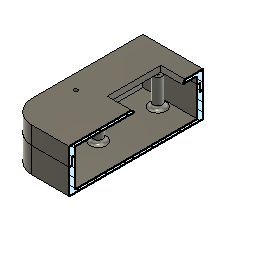
ReceiverCase (Autodesk Fusion 360 design; units mm, degrees)
Autodesk Fusion 360 part; units mm, degrees
sketch "Sketch1" plane through (0, 0, 0) normal (0, 1, 0) x (1, 0, 0)
  line L0 (22.5, 22.5) -> (-22.5, 22.5)
  line L1 (-22.5, 22.5) -> (-22.5, -22.5)
  line L2 (-22.5, -22.5) -> (22.5, -22.5)
  line L3 (22.5, -22.5) -> (22.5, 22.5)
  line L4 (22.5, 22.5) -> (-22.5, -22.5) construction
  line L5 (-22.5, 22.5) -> (22.5, -22.5) construction
  circle A0 centre (-20, 20) radius 1
  circle A1 centre (20, 20) radius 1
  circle A2 centre (20, -20) radius 1
  circle A3 centre (-20, -20) radius 1
  line L6 (-13.9694, -16) -> (-13.9694, 16)
  line L7 (-13.9694, 16) -> (7.9088, 16)
  line L8 (7.9088, 16) -> (7.9088, -16)
  line L9 (7.9088, -16) -> (-13.9694, -16)
  line L10 (25, -29.5) -> (-25, -29.5)
  line L11 (-25, -29.5) -> (-25, -54.5)
  line L12 (-25, -54.5) -> (25, -54.5)
  line L13 (25, -54.5) -> (25, -29.5)
  line L14 (25, -29.5) -> (-25, -54.5) construction
  line L15 (-25, -29.5) -> (25, -54.5) construction
  line L16 (30, 30) -> (-40, 30)
  line L17 (-40, 30) -> (-40, -60)
  line L18 (-40, -60) -> (30, -60)
  line L19 (30, -60) -> (30, 30)
  arc A4 (30, 22.5) -> (22.5, 30) centre (22.5, 22.5) ccw
  arc A5 (-40, -44) -> (-25, -60) centre (-23.9667, -44) ccw
  arc A6 (25, -60) -> (30, -55) centre (25, -55) ccw
  circle A7 centre (-20, 20) radius 3
  circle A8 centre (20, 20) radius 3
  circle A9 centre (20, -20) radius 3
  circle A10 centre (-20, -20) radius 3
  dimension "d1" = 45
  dimension "d2" = 45
  dimension "d9" = 50
  dimension "d10" = 25
extrude "Extrude1" add sketch "Sketch1" along normal blind 1 contours L0 L3 A8 | L0 L3 A8 | L0 L1 L2 L3 A7 A8 A9 A10 | L0 L1 A7 | L2 L3 A9 | L0 L1 A7 | L2 L3 A9 | L1 L2 A10 | L1 L2 A10 | L6 L7 L8 L9 makes body 1
extrude "Extrude2" add sketch "Sketch1" along normal blind 6 contours L6 L7 L8 L9 bodies 1
extrude "Extrude3" add sketch "Sketch1" along normal blind 20 separate body contours L10 L11 L12 L13 makes body 2
sketch "Sketch2" plane through (0, 0, 0) normal (0, 1, 0) x (1, 0, 0)
  arc A0 (30, 22.5) -> (22.5, 30) centre (22.5, 22.5) ccw
  line L0 (-40, 30) -> (22.5, 30)
  line L1 (30, 22.5) -> (30, -55)
  arc A1 (25, -60) -> (30, -55) centre (25, -55) ccw
  line L2 (-25, -60) -> (25, -60)
  line L3 (-40, 30) -> (-40, -44)
  line L4 (-38, 28) -> (22.5, 28)
  arc A2 (28, 22.5) -> (22.5, 28) centre (22.5, 22.5) ccw
  line L5 (28, 22.5) -> (28, -55)
  arc A3 (25, -58) -> (28, -55) centre (25, -55) ccw
  line L6 (-24.1692, -58) -> (25, -58)
  line L7 (-38, 28) -> (-38, -43.2439)
  line L8 (26, 22.5) -> (26, -55)
  arc A4 (25, -56) -> (26, -55) centre (25, -55) ccw
  line L9 (-23.3355, -56) -> (25, -56)
  line L10 (-36, 26) -> (-36, -42.4854)
  line L11 (-36, 26) -> (22.5, 26)
  arc A5 (26, 22.5) -> (22.5, 26) centre (22.5, 22.5) ccw
  arc A6 (-40, -44) -> (-25, -60) centre (-23.9667, -44) ccw
  arc A7 (-38, -43.2439) -> (-24.1692, -58) centre (-23.213, -43.2439) ccw
  arc A8 (-36, -42.4854) -> (-23.3355, -56) centre (-22.4569, -42.4854) ccw
  circle A9 centre (-30, -25) radius 3
extrude "Extrude4" add sketch "Sketch2" against normal blind 2 separate body contours A0 L0 L1 A1 L2 L3 A6 | L4 A2 L5 A3 L6 L7 A7 | L8 A4 L9 L10 L11 A5 A8 | A9 makes body 3
extrude "Extrude5" add sketch "Sketch2" along normal blind 15 contours A0 L0 L1 A1 L2 L3 A6 | L4 A2 L5 A3 L6 L7 A7 bodies 3
extrude "Extrude6" add sketch "Sketch2" along normal blind 20 contours L4 A2 L5 A3 L6 L7 A7 bodies 3
extrude "Extrude7" add sketch "Sketch2" along normal blind 25 and the other way blind -15 separate body contours A0 L0 L1 A1 L2 L3 A6 makes body 4
extrude "Extrude8" add sketch "Sketch2" along normal blind 25 and the other way blind -20 contours A0 L0 L1 A1 L2 L3 A6 | L4 A2 L5 A3 L6 L7 A7 bodies 4
extrude "Extrude9" add sketch "Sketch2" along normal blind 25 and the other way blind -27 contours A0 L0 L1 A1 L2 L3 A6 | L4 A2 L5 A3 L6 L7 A7 | L8 A4 L9 L10 L11 A5 A8 | A9 bodies 4
extrude "Extrude10" cut sketch "Sketch1" along normal blind 50 contours L6 L7 L8 L9 bodies 4
chamfer "Chamfer1" distance 2 angle 45 4 edges at (-3.0303, 27, 16) (-13.9694, 27, 0) (7.9088, 27, 0) (-3.0303, 27, -16) on bodies 4
hole "Hole1" at (-29.7102, 12.9727, -30) direction (0, 0, 1) diameter 7 depth 19 tip angle 118 bodies 3 4
hole "Hole2" at (-29.7102, 12.9727, -26) direction (0, 0, -1) diameter 11 depth 2 tip angle 180 bodies 3
move_body "Move1" bodies 1 to x (1, 0, 0) y (0, 1, 0) z (0, 0, 1) at (0, 19, 0)
move_body "Move2" bodies 2 to x (1, 0, 0) y (0, 1, 0) z (0, 0, 1) at (0, 3, 0)
extrude "Extrude11" add sketch "Sketch1" along normal blind 19 contours L0 L3 A8 | L0 A8 | L3 A8 | L0 L1 A7 | L0 A7 | L3 A9 | L2 L3 A9 | L2 A9 | L1 A7 | L2 A10 | L1 L2 A10 | L1 A10 | A0 | A1 | A2 | A3 picked at (19.9751, 21.9991) picked at (-19.9751, 21.9991) picked at (19.9751, -21.9991) picked at (-19.9751, -21.9991) bodies 3
extrude "Extrude12" add sketch "Sketch1" along normal blind 22 contours A0 | A1 | A2 | A3 bodies 3
fillet "Fillet1" radius 2.5 4 edges at (-22.797, 0, 18.9152) (-22.797, 0, -21.0848) (17.203, 0, 18.9152) (17.203, 0, -21.0848) on bodies 3
sketch "Sketch3" plane through (-36, 0, 0) normal (1, 0, 0) x (0, 0, -1)
  line L0 (-42.4854, 0) -> (26, 0)
  line L1 (26, 0) -> (26, 20)
  line L2 (26, 20) -> (-42.4854, 20)
  line L3 (-42.4854, 20) -> (-42.4854, 0)
  line L4 (-6, 8) -> (5, 8)
  line L5 (5, 8) -> (5, 0)
  line L6 (5, 0) -> (-6, 0)
  line L7 (-6, 0) -> (-6, 8)
extrude "Extrude13" cut sketch "Sketch3" against normal blind 6 contours L0 L4 L5 L6 L7 bodies 3
chamfer "Chamfer2" distance 2 angle 45 2 edges at (-38, 8, -5) (-38, 8, 6) on bodies 3
extrude "Extrude15" add sketch "Sketch2" along normal blind 25 contours A9 bodies 3
hole "Hole4" at (-29.9997, 27, 24.9995) direction (0, -1, 0) diameter 2.4 depth 15 tip angle 90 bodies 3 4
hidden bodies 1 2
named bodies: "screen", "psu", "bottom", "top"
